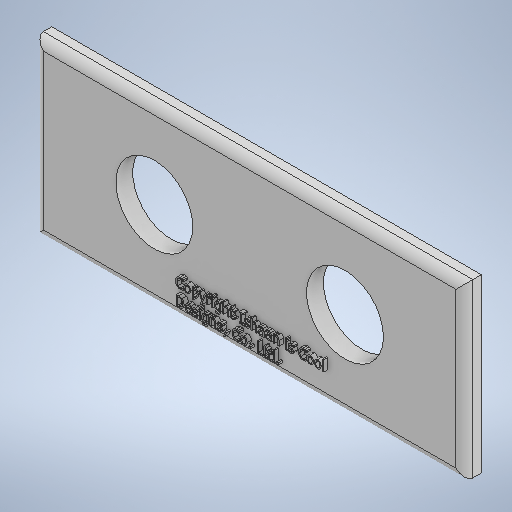
# Autodesk Inventor part: Hole Position Test Plate
Saved by Autodesk Inventor 2025.1 (Build 291241000, 241)
## iProperties
Created: 2024-12-13
Part Number: Hole Position Test Plate
Material: Generic
Document SubType Name: Modeling
Designer: ishaa
Density: 1 g/cm^3
Appearance: Default
Author: ishaa
Autodesk Inventor part; units mm, degrees
ref_plane "YZ Plane" through (0, 0, 0) normal (1, 0, 0) x (0, 1, 0)
ref_plane "XZ Plane" through (0, 0, 0) normal (0, 1, 0) x (-1, 0, 0)
ref_plane "XY Plane" through (0, 0, 0) normal (0, 0, 1) x (1, 0, 0)
sketch "Sketch1" plane through (0, 0, 0) normal (0, 0, 1) x (1, 0, 0)
  line L0 (-25.4, -10.16) -> (25.4, -10.16)
  line L1 (25.4, -10.16) -> (25.4, 10.16)
  line L2 (25.4, 10.16) -> (-25.4, 10.16)
  line L3 (-25.4, 10.16) -> (-25.4, -10.16)
  line L4 (-25.4, -10.16) -> (25.4, 10.16) construction
  line L5 (25.4, -10.16) -> (-25.4, 10.16) construction
  circle A0 centre (-11.276, 0) radius 4.55
  circle A1 centre (11.276, 0) radius 4.55
  line L6 (-11.276, 0) -> (11.276, 0) construction
  line L7 (0, 0) -> (0, 7.6048) construction
  line L8 (0, 15.995) -> (0, -21.9957) construction
  dimension "d0" = 50.8
  dimension "d1" = 20.32
  dimension "d2" = 9.1
  dimension "d3" = 9.1
  dimension "d4" = 22.552
  constraints: 18 end point, 3 midpoint, 3 vertical, 2 centre point, 2 horizontal, 2 parallel, 1 collinear, 1 perpendicular
  measures "d0" distance of L2.end L1.end
  measures "d1" distance of L1.end L0.end
  measures "d2" diameter of A0
  measures "d3" diameter of A1
  measures "d4" distance of L6.end L6.start
extrude "Extrusion1" add sketch "Sketch1" along normal blind 2
sketch "Sketch2" plane through (0, 0, 2) normal (0, 0, 1) x (1, 0, 0)
  line L0 (-8.3124, -5.381) -> (11.7699, -5.381) construction
  line L1 (11.7699, -5.381) -> (11.7699, -6.9151) construction
  line L2 (11.7699, -6.9151) -> (-8.3124, -6.9151) construction
  line L3 (-8.3124, -6.9151) -> (-8.3124, -5.381) construction
  spline S0 degree 2 poles (-7.7232, -6.6536) (-7.8397, -6.6536) (-8.0367, -6.575) (-8.1086, -6.4963) knots 0 0 0 1 2 2 2
  spline S1 degree 2 poles (-8.1086, -6.4963) (-8.1804, -6.4187) (-8.259, -6.1857) (-8.259, -6.0343) knots 0 0 0 1 2 2 2
  spline S2 degree 2 poles (-8.259, -6.0343) (-8.259, -5.8838) (-8.1823, -5.6606) (-8.1095, -5.578) knots 0 0 0 1 2 2 2
  spline S3 degree 2 poles (-8.1095, -5.578) (-8.0377, -5.4975) (-7.8416, -5.413) (-7.7203, -5.413) knots 0 0 0 1 2 2 2
  spline S4 degree 2 poles (-7.7203, -5.413) (-7.6601, -5.413) (-7.5543, -5.4305) (-7.5096, -5.4441) knots 0 0 0 1 2 2 2
  spline S5 degree 2 poles (-7.5096, -5.4441) (-7.4708, -5.4567) (-7.3902, -5.4926) (-7.3504, -5.514) knots 0 0 0 1 2 2 2
  line L4 (-7.3504, -5.514) -> (-7.3504, -5.7062)
  line L5 (-7.3504, -5.7062) -> (-7.3631, -5.7062)
  spline S6 degree 2 poles (-7.3631, -5.7062) (-7.3844, -5.6868) (-7.4504, -5.6324) (-7.498, -5.6062) knots 0 0 0 1 2 2 2
  spline S7 degree 2 poles (-7.498, -5.6062) (-7.5436, -5.581) (-7.6514, -5.5489) (-7.7213, -5.5489) knots 0 0 0 1 2 2 2
  spline S8 degree 2 poles (-7.7213, -5.5489) (-7.7979, -5.5489) (-7.9348, -5.612) (-7.9863, -5.6722) knots 0 0 0 1 2 2 2
  spline S9 degree 2 poles (-7.9863, -5.6722) (-8.0367, -5.7334) (-8.093, -5.9188) (-8.093, -6.0343) knots 0 0 0 1 2 2 2
  spline S10 degree 2 poles (-8.093, -6.0343) (-8.093, -6.1576) (-8.0338, -6.3352) (-7.9824, -6.3964) knots 0 0 0 1 2 2 2
  spline S11 degree 2 poles (-7.9824, -6.3964) (-7.9319, -6.4556) (-7.797, -6.5158) (-7.7213, -6.5158) knots 0 0 0 1 2 2 2
  spline S12 degree 2 poles (-7.7213, -6.5158) (-7.6523, -6.5158) (-7.5349, -6.4818) (-7.4893, -6.4565) knots 0 0 0 1 2 2 2
  spline S13 degree 2 poles (-7.4893, -6.4565) (-7.4456, -6.4313) (-7.3805, -6.3789) (-7.3621, -6.3604) knots 0 0 0 1 2 2 2
  line L6 (-7.3621, -6.3604) -> (-7.3504, -6.3604)
  line L7 (-7.3504, -6.3604) -> (-7.3504, -6.5507)
  spline S14 degree 2 poles (-7.3504, -6.5507) (-7.3902, -6.5692) (-7.4601, -6.6031) (-7.5096, -6.6187) knots 0 0 0 1 2 2 2
  spline S15 degree 2 poles (-7.5096, -6.6187) (-7.5621, -6.6361) (-7.6514, -6.6536) (-7.7232, -6.6536) knots 0 0 0 1 2 2 2
  spline S16 degree 2 poles (-6.4749, -6.1828) (-6.4749, -6.41) (-6.6933, -6.6575) (-6.8758, -6.6575) knots 0 0 0 1 2 2 2
  spline S17 degree 2 poles (-6.8758, -6.6575) (-7.0631, -6.6575) (-7.2776, -6.4022) (-7.2776, -6.1828) knots 0 0 0 1 2 2 2
  spline S18 degree 2 poles (-7.2776, -6.1828) (-7.2776, -5.9576) (-7.0563, -5.7081) (-6.8758, -5.7081) knots 0 0 0 1 2 2 2
  spline S19 degree 2 poles (-6.8758, -5.7081) (-6.6933, -5.7081) (-6.4749, -5.9566) (-6.4749, -6.1828) knots 0 0 0 1 2 2 2
  spline S20 degree 2 poles (-6.6311, -6.1828) (-6.6311, -6.0081) (-6.7583, -5.8382) (-6.8758, -5.8382) knots 0 0 0 1 2 2 2
  spline S21 degree 2 poles (-6.8758, -5.8382) (-6.9932, -5.8382) (-7.1214, -6.0081) (-7.1214, -6.1828) knots 0 0 0 1 2 2 2
  spline S22 degree 2 poles (-7.1214, -6.1828) (-7.1214, -6.3527) (-6.9932, -6.5274) (-6.8758, -6.5274) knots 0 0 0 1 2 2 2
  spline S23 degree 2 poles (-6.8758, -6.5274) (-6.7593, -6.5274) (-6.6311, -6.3556) (-6.6311, -6.1828) knots 0 0 0 1 2 2 2
  spline S24 degree 2 poles (-5.5663, -6.1585) (-5.5663, -6.3837) (-5.7808, -6.6497) (-5.9448, -6.6497) knots 0 0 0 1 2 2 2
  spline S25 degree 2 poles (-5.9448, -6.6497) (-6.0118, -6.6497) (-6.1147, -6.6187) (-6.1681, -6.5866) knots 0 0 0 1 2 2 2
  line L8 (-6.1681, -6.5866) -> (-6.1681, -6.9633)
  line L9 (-6.1681, -6.9633) -> (-6.3195, -6.9633)
  line L10 (-6.3195, -6.9633) -> (-6.3195, -5.7334)
  line L11 (-6.3195, -5.7334) -> (-6.1681, -5.7334)
  line L12 (-6.1681, -5.7334) -> (-6.1681, -5.8275)
  spline S26 degree 2 poles (-6.1681, -5.8275) (-6.1118, -5.7761) (-5.974, -5.7081) (-5.8934, -5.7081) knots 0 0 0 1 2 2 2
  spline S27 degree 2 poles (-5.8934, -5.7081) (-5.7391, -5.7081) (-5.5663, -5.9527) (-5.5663, -6.1585) knots 0 0 0 1 2 2 2
  spline S28 degree 2 poles (-5.7225, -6.176) (-5.7225, -6.0217) (-5.8206, -5.8518) (-5.9303, -5.8518) knots 0 0 0 1 2 2 2
  spline S29 degree 2 poles (-5.9303, -5.8518) (-5.9943, -5.8518) (-6.1147, -5.9091) (-6.1681, -5.9537) knots 0 0 0 1 2 2 2
  line L13 (-6.1681, -5.9537) -> (-6.1681, -6.4643)
  spline S30 degree 2 poles (-6.1681, -6.4643) (-6.1089, -6.4925) (-6.0244, -6.5138) (-5.9701, -6.5138) knots 0 0 0 1 2 2 2
  spline S31 degree 2 poles (-5.9701, -6.5138) (-5.8526, -6.5138) (-5.7225, -6.341) (-5.7225, -6.176) knots 0 0 0 1 2 2 2
  line L14 (-4.7033, -5.7334) -> (-5.1867, -6.9633)
  line L15 (-5.1867, -6.9633) -> (-5.3488, -6.9633)
  line L16 (-5.3488, -6.9633) -> (-5.1877, -6.5886)
  line L17 (-5.1877, -6.5886) -> (-5.5138, -5.7334)
  line L18 (-5.5138, -5.7334) -> (-5.3508, -5.7334)
  line L19 (-5.3508, -5.7334) -> (-5.1052, -6.3993)
  line L20 (-5.1052, -6.3993) -> (-4.8606, -5.7334)
  line L21 (-4.8606, -5.7334) -> (-4.7033, -5.7334)
  line L22 (-4.1121, -5.8955) -> (-4.1199, -5.8955)
  spline S32 degree 2 poles (-4.1199, -5.8955) (-4.1374, -5.8906) (-4.1752, -5.8887) (-4.2014, -5.8887) knots 0 0 0 1 2 2 2
  spline S33 degree 2 poles (-4.2014, -5.8887) (-4.2626, -5.8887) (-4.383, -5.9421) (-4.4373, -5.9945) knots 0 0 0 1 2 2 2
  line L23 (-4.4373, -5.9945) -> (-4.4373, -6.6322)
  line L24 (-4.4373, -6.6322) -> (-4.5888, -6.6322)
  line L25 (-4.5888, -6.6322) -> (-4.5888, -5.7334)
  line L26 (-4.5888, -5.7334) -> (-4.4373, -5.7334)
  line L27 (-4.4373, -5.7334) -> (-4.4373, -5.8673)
  spline S34 degree 2 poles (-4.4373, -5.8673) (-4.3548, -5.7935) (-4.2315, -5.7334) (-4.1733, -5.7334) knots 0 0 0 1 2 2 2
  spline S35 degree 2 poles (-4.1733, -5.7334) (-4.15, -5.7334) (-4.1267, -5.7353) (-4.1121, -5.7382) knots 0 0 0 1 2 2 2
  line L28 (-4.1121, -5.7382) -> (-4.1121, -5.8955)
  line L29 (-3.8403, -6.6322) -> (-3.9918, -6.6322)
  line L30 (-3.9918, -6.6322) -> (-3.9918, -5.7334)
  line L31 (-3.9918, -5.7334) -> (-3.8403, -5.7334)
  line L32 (-3.8403, -5.7334) -> (-3.8403, -6.6322)
  line L33 (-3.8297, -5.5839) -> (-4.0015, -5.5839)
  line L34 (-4.0015, -5.5839) -> (-4.0015, -5.4266)
  line L35 (-4.0015, -5.4266) -> (-3.8297, -5.4266)
  line L36 (-3.8297, -5.4266) -> (-3.8297, -5.5839)
  spline S36 degree 2 poles (-3.586, -6.7759) (-3.5705, -6.7827) (-3.5113, -6.8041) (-3.4734, -6.8128) knots 0 0 0 1 2 2 2
  spline S37 degree 2 poles (-3.4734, -6.8128) (-3.4317, -6.8235) (-3.3608, -6.8361) (-3.3191, -6.8361) knots 0 0 0 1 2 2 2
  spline S38 degree 2 poles (-3.3191, -6.8361) (-3.2492, -6.8361) (-3.1521, -6.7992) (-3.1249, -6.7662) knots 0 0 0 1 2 2 2
  spline S39 degree 2 poles (-3.1249, -6.7662) (-3.0987, -6.7332) (-3.0783, -6.6468) (-3.0783, -6.5915) knots 0 0 0 1 2 2 2
  line L37 (-3.0783, -6.5915) -> (-3.0783, -6.5128)
  spline S40 degree 2 poles (-3.0783, -6.5128) (-3.1395, -6.5662) (-3.2569, -6.6167) (-3.3453, -6.6167) knots 0 0 0 1 2 2 2
  spline S41 degree 2 poles (-3.3453, -6.6167) (-3.4986, -6.6167) (-3.6802, -6.3886) (-3.6802, -6.1741) knots 0 0 0 1 2 2 2
  spline S42 degree 2 poles (-3.6802, -6.1741) (-3.6802, -6.0624) (-3.6171, -5.8896) (-3.5646, -5.8285) knots 0 0 0 1 2 2 2
  spline S43 degree 2 poles (-3.5646, -5.8285) (-3.5142, -5.7712) (-3.3754, -5.7081) (-3.3016, -5.7081) knots 0 0 0 1 2 2 2
  spline S44 degree 2 poles (-3.3016, -5.7081) (-3.2317, -5.7081) (-3.1298, -5.7411) (-3.0783, -5.7712) knots 0 0 0 1 2 2 2
  line L38 (-3.0783, -5.7712) -> (-3.0696, -5.7334)
  line L39 (-3.0696, -5.7334) -> (-2.9269, -5.7334)
  line L40 (-2.9269, -5.7334) -> (-2.9269, -6.5294)
  spline S45 degree 2 poles (-2.9269, -6.5294) (-2.9269, -6.7584) (-3.1259, -6.972) (-3.3307, -6.972) knots 0 0 0 1 2 2 2
  spline S46 degree 2 poles (-3.3307, -6.972) (-3.3967, -6.972) (-3.5346, -6.9506) (-3.5938, -6.9332) knots 0 0 0 1 2 2 2
  line L41 (-3.5938, -6.9332) -> (-3.5938, -6.7759)
  line L42 (-3.5938, -6.7759) -> (-3.586, -6.7759)
  line L43 (-3.0783, -6.3886) -> (-3.0783, -5.8945)
  spline S47 degree 2 poles (-3.0783, -5.8945) (-3.1346, -5.8673) (-3.2297, -5.844) (-3.2773, -5.844) knots 0 0 0 1 2 2 2
  spline S48 degree 2 poles (-3.2773, -5.844) (-3.3919, -5.844) (-3.5239, -6.0129) (-3.5239, -6.1712) knots 0 0 0 1 2 2 2
  spline S49 degree 2 poles (-3.5239, -6.1712) (-3.5239, -6.3206) (-3.4239, -6.4769) (-3.3113, -6.4769) knots 0 0 0 1 2 2 2
  spline S50 degree 2 poles (-3.3113, -6.4769) (-3.2521, -6.4769) (-3.1278, -6.4303) (-3.0783, -6.3886) knots 0 0 0 1 2 2 2
  line L44 (-2.0018, -6.6322) -> (-2.1532, -6.6322)
  line L45 (-2.1532, -6.6322) -> (-2.1532, -6.1197)
  spline S51 degree 2 poles (-2.1532, -6.1197) (-2.1532, -6.0576) (-2.1649, -5.9508) (-2.1823, -5.9188) knots 0 0 0 1 2 2 2
  spline S52 degree 2 poles (-2.1823, -5.9188) (-2.2008, -5.8848) (-2.2668, -5.8518) (-2.3231, -5.8518) knots 0 0 0 1 2 2 2
  spline S53 degree 2 poles (-2.3231, -5.8518) (-2.3794, -5.8518) (-2.4988, -5.912) (-2.5561, -5.9605) knots 0 0 0 1 2 2 2
  line L46 (-2.5561, -5.9605) -> (-2.5561, -6.6322)
  line L47 (-2.5561, -6.6322) -> (-2.7075, -6.6322)
  line L48 (-2.7075, -6.6322) -> (-2.7075, -5.381)
  line L49 (-2.7075, -5.381) -> (-2.5561, -5.381)
  line L50 (-2.5561, -5.381) -> (-2.5561, -5.8333)
  spline S54 degree 2 poles (-2.5561, -5.8333) (-2.4881, -5.7722) (-2.3571, -5.7081) (-2.2833, -5.7081) knots 0 0 0 1 2 2 2
  spline S55 degree 2 poles (-2.2833, -5.7081) (-2.1513, -5.7081) (-2.0018, -5.8829) (-2.0018, -6.0488) knots 0 0 0 1 2 2 2
  line L51 (-2.0018, -6.0488) -> (-2.0018, -6.6322)
  spline S56 degree 2 poles (-1.5174, -6.6497) (-1.6407, -6.6497) (-1.7795, -6.509) (-1.7795, -6.3566) knots 0 0 0 1 2 2 2
  line L52 (-1.7795, -6.3566) -> (-1.7795, -5.8586)
  line L53 (-1.7795, -5.8586) -> (-1.8814, -5.8586)
  line L54 (-1.8814, -5.8586) -> (-1.8814, -5.7334)
  line L55 (-1.8814, -5.7334) -> (-1.7795, -5.7334)
  line L56 (-1.7795, -5.7334) -> (-1.7795, -5.4752)
  line L57 (-1.7795, -5.4752) -> (-1.6281, -5.4752)
  line L58 (-1.6281, -5.4752) -> (-1.6281, -5.7334)
  line L59 (-1.6281, -5.7334) -> (-1.3495, -5.7334)
  line L60 (-1.3495, -5.7334) -> (-1.3495, -5.8586)
  line L61 (-1.3495, -5.8586) -> (-1.6281, -5.8586)
  line L62 (-1.6281, -5.8586) -> (-1.6281, -6.2867)
  spline S57 degree 2 poles (-1.6281, -6.2867) (-1.6281, -6.3546) (-1.6232, -6.4294) (-1.6067, -6.4614) knots 0 0 0 1 2 2 2
  spline S58 degree 2 poles (-1.6067, -6.4614) (-1.5931, -6.4896) (-1.532, -6.5177) (-1.4795, -6.5177) knots 0 0 0 1 2 2 2
  spline S59 degree 2 poles (-1.4795, -6.5177) (-1.4427, -6.5177) (-1.3737, -6.4954) (-1.3582, -6.4886) knots 0 0 0 1 2 2 2
  line L63 (-1.3582, -6.4886) -> (-1.3495, -6.4886)
  line L64 (-1.3495, -6.4886) -> (-1.3495, -6.6245)
  spline S60 degree 2 poles (-1.3495, -6.6245) (-1.3922, -6.6361) (-1.4795, -6.6497) (-1.5174, -6.6497) knots 0 0 0 1 2 2 2
  line L65 (-0.2943, -6.6322) -> (-0.7583, -6.6322)
  line L66 (-0.7583, -6.6322) -> (-0.7583, -6.5099)
  line L67 (-0.7583, -6.5099) -> (-0.6059, -6.5099)
  line L68 (-0.6059, -6.5099) -> (-0.6059, -5.5567)
  line L69 (-0.6059, -5.5567) -> (-0.7583, -5.5567)
  line L70 (-0.7583, -5.5567) -> (-0.7583, -5.4344)
  line L71 (-0.7583, -5.4344) -> (-0.2943, -5.4344)
  line L72 (-0.2943, -5.4344) -> (-0.2943, -5.5567)
  line L73 (-0.2943, -5.5567) -> (-0.4467, -5.5567)
  line L74 (-0.4467, -5.5567) -> (-0.4467, -6.5099)
  line L75 (-0.4467, -6.5099) -> (-0.2943, -6.5099)
  line L76 (-0.2943, -6.5099) -> (-0.2943, -6.6322)
  spline S61 degree 2 poles (0.1338, -6.6536) (0.0435, -6.6536) (-0.1128, -6.6051) (-0.1642, -6.5779) knots 0 0 0 1 2 2 2
  line L77 (-0.1642, -6.5779) -> (-0.1642, -6.408)
  line L78 (-0.1642, -6.408) -> (-0.1565, -6.408)
  spline S62 degree 2 poles (-0.1565, -6.408) (-0.137, -6.4235) (-0.0846, -6.4604) (-0.0409, -6.4808) knots 0 0 0 1 2 2 2
  spline S63 degree 2 poles (-0.0409, -6.4808) (-0.0031, -6.4993) (0.0901, -6.5264) (0.1396, -6.5264) knots 0 0 0 1 2 2 2
  spline S64 degree 2 poles (0.1396, -6.5264) (0.1755, -6.5264) (0.258, -6.5099) (0.2774, -6.4963) knots 0 0 0 1 2 2 2
  spline S65 degree 2 poles (0.2774, -6.4963) (0.3056, -6.4779) (0.3308, -6.4362) (0.3308, -6.3935) knots 0 0 0 1 2 2 2
  spline S66 degree 2 poles (0.3308, -6.3935) (0.3308, -6.3401) (0.2726, -6.2847) (0.1979, -6.2663) knots 0 0 0 1 2 2 2
  spline S67 degree 2 poles (0.1979, -6.2663) (0.1687, -6.2595) (0.0755, -6.2401) (0.0357, -6.2294) knots 0 0 0 1 2 2 2
  spline S68 degree 2 poles (0.0357, -6.2294) (-0.0672, -6.1993) (-0.1603, -6.0751) (-0.1603, -5.9867) knots 0 0 0 1 2 2 2
  spline S69 degree 2 poles (-0.1603, -5.9867) (-0.1603, -5.8644) (0.0231, -5.712) (0.1746, -5.712) knots 0 0 0 1 2 2 2
  spline S70 degree 2 poles (0.1746, -5.712) (0.2493, -5.712) (0.4007, -5.7489) (0.4522, -5.777) knots 0 0 0 1 2 2 2
  line L79 (0.4522, -5.777) -> (0.4522, -5.9392)
  line L80 (0.4522, -5.9392) -> (0.4444, -5.9392)
  spline S71 degree 2 poles (0.4444, -5.9392) (0.3862, -5.8926) (0.2444, -5.8392) (0.1716, -5.8392) knots 0 0 0 1 2 2 2
  spline S72 degree 2 poles (0.1716, -5.8392) (0.0969, -5.8392) (-0.006, -5.9023) (-0.006, -5.9654) knots 0 0 0 1 2 2 2
  spline S73 degree 2 poles (-0.006, -5.9654) (-0.006, -6.0226) (0.0552, -6.078) (0.1231, -6.0954) knots 0 0 0 1 2 2 2
  spline S74 degree 2 poles (0.1231, -6.0954) (0.1561, -6.1042) (0.2396, -6.1217) (0.2852, -6.1323) knots 0 0 0 1 2 2 2
  spline S75 degree 2 poles (0.2852, -6.1323) (0.3842, -6.1576) (0.4852, -6.2731) (0.4852, -6.3731) knots 0 0 0 1 2 2 2
  spline S76 degree 2 poles (0.4852, -6.3731) (0.4852, -6.4313) (0.4396, -6.5342) (0.3949, -6.5721) knots 0 0 0 1 2 2 2
  spline S77 degree 2 poles (0.3949, -6.5721) (0.3473, -6.6119) (0.226, -6.6536) (0.1338, -6.6536) knots 0 0 0 1 2 2 2
  line L81 (1.3316, -6.6322) -> (1.1802, -6.6322)
  line L82 (1.1802, -6.6322) -> (1.1802, -6.1197)
  spline S78 degree 2 poles (1.1802, -6.1197) (1.1802, -6.0576) (1.1686, -5.9508) (1.1511, -5.9188) knots 0 0 0 1 2 2 2
  spline S79 degree 2 poles (1.1511, -5.9188) (1.1327, -5.8848) (1.0666, -5.8518) (1.0103, -5.8518) knots 0 0 0 1 2 2 2
  spline S80 degree 2 poles (1.0103, -5.8518) (0.954, -5.8518) (0.8346, -5.912) (0.7774, -5.9605) knots 0 0 0 1 2 2 2
  line L83 (0.7774, -5.9605) -> (0.7774, -6.6322)
  line L84 (0.7774, -6.6322) -> (0.6259, -6.6322)
  line L85 (0.6259, -6.6322) -> (0.6259, -5.381)
  line L86 (0.6259, -5.381) -> (0.7774, -5.381)
  line L87 (0.7774, -5.381) -> (0.7774, -5.8333)
  spline S81 degree 2 poles (0.7774, -5.8333) (0.8453, -5.7722) (0.9764, -5.7081) (1.0501, -5.7081) knots 0 0 0 1 2 2 2
  spline S82 degree 2 poles (1.0501, -5.7081) (1.1822, -5.7081) (1.3316, -5.8829) (1.3316, -6.0488) knots 0 0 0 1 2 2 2
  line L88 (1.3316, -6.0488) -> (1.3316, -6.6322)
  spline S83 degree 2 poles (2.0451, -6.5371) (2.0267, -6.5507) (1.9646, -6.5992) (1.9354, -6.6138) knots 0 0 0 1 2 2 2
  spline S84 degree 2 poles (1.9354, -6.6138) (1.8956, -6.6352) (1.8209, -6.6575) (1.7529, -6.6575) knots 0 0 0 1 2 2 2
  spline S85 degree 2 poles (1.7529, -6.6575) (1.6976, -6.6575) (1.5976, -6.6157) (1.5598, -6.5779) knots 0 0 0 1 2 2 2
  spline S86 degree 2 poles (1.5598, -6.5779) (1.5238, -6.541) (1.4802, -6.4323) (1.4802, -6.3721) knots 0 0 0 1 2 2 2
  spline S87 degree 2 poles (1.4802, -6.3721) (1.4802, -6.2789) (1.5588, -6.1469) (1.6442, -6.109) knots 0 0 0 1 2 2 2
  spline S88 degree 2 poles (1.6442, -6.109) (1.7199, -6.0741) (1.9257, -6.0479) (2.0451, -6.0411) knots 0 0 0 1 2 2 2
  line L89 (2.0451, -6.0411) -> (2.0451, -6.012)
  spline S89 degree 2 poles (2.0451, -6.012) (2.0451, -5.9595) (2.0131, -5.8945) (1.984, -5.8761) knots 0 0 0 1 2 2 2
  spline S90 degree 2 poles (1.984, -5.8761) (1.9548, -5.8576) (1.8714, -5.846) (1.8267, -5.846) knots 0 0 0 1 2 2 2
  spline S91 degree 2 poles (1.8267, -5.846) (1.7743, -5.846) (1.6326, -5.877) (1.5617, -5.9071) knots 0 0 0 1 2 2 2
  line L90 (1.5617, -5.9071) -> (1.553, -5.9071)
  line L91 (1.553, -5.9071) -> (1.553, -5.7528)
  spline S92 degree 2 poles (1.553, -5.7528) (1.5947, -5.7411) (1.751, -5.712) (1.8277, -5.712) knots 0 0 0 1 2 2 2
  spline S93 degree 2 poles (1.8277, -5.712) (1.9209, -5.712) (2.048, -5.7411) (2.0985, -5.779) knots 0 0 0 1 2 2 2
  spline S94 degree 2 poles (2.0985, -5.779) (2.148, -5.8159) (2.1966, -5.9333) (2.1966, -6.0178) knots 0 0 0 1 2 2 2
  line L92 (2.1966, -6.0178) -> (2.1966, -6.6322)
  line L93 (2.1966, -6.6322) -> (2.0451, -6.6322)
  line L94 (2.0451, -6.6322) -> (2.0451, -6.5371)
  line L95 (2.0451, -6.4109) -> (2.0451, -6.1615)
  spline S95 degree 2 poles (2.0451, -6.1615) (1.9908, -6.1663) (1.8267, -6.1828) (1.7753, -6.1983) knots 0 0 0 1 2 2 2
  spline S96 degree 2 poles (1.7753, -6.1983) (1.7151, -6.2168) (1.6365, -6.2935) (1.6365, -6.3614) knots 0 0 0 1 2 2 2
  spline S97 degree 2 poles (1.6365, -6.3614) (1.6365, -6.4391) (1.7238, -6.5177) (1.8073, -6.5177) knots 0 0 0 1 2 2 2
  spline S98 degree 2 poles (1.8073, -6.5177) (1.8782, -6.5177) (1.9946, -6.4565) (2.0451, -6.4109) knots 0 0 0 1 2 2 2
  spline S99 degree 2 poles (2.91, -6.5371) (2.8916, -6.5507) (2.8295, -6.5992) (2.8003, -6.6138) knots 0 0 0 1 2 2 2
  spline S100 degree 2 poles (2.8003, -6.6138) (2.7605, -6.6352) (2.6858, -6.6575) (2.6178, -6.6575) knots 0 0 0 1 2 2 2
  spline S101 degree 2 poles (2.6178, -6.6575) (2.5625, -6.6575) (2.4625, -6.6157) (2.4247, -6.5779) knots 0 0 0 1 2 2 2
  spline S102 degree 2 poles (2.4247, -6.5779) (2.3888, -6.541) (2.3451, -6.4323) (2.3451, -6.3721) knots 0 0 0 1 2 2 2
  spline S103 degree 2 poles (2.3451, -6.3721) (2.3451, -6.2789) (2.4237, -6.1469) (2.5091, -6.109) knots 0 0 0 1 2 2 2
  spline S104 degree 2 poles (2.5091, -6.109) (2.5848, -6.0741) (2.7906, -6.0479) (2.91, -6.0411) knots 0 0 0 1 2 2 2
  line L96 (2.91, -6.0411) -> (2.91, -6.012)
  spline S105 degree 2 poles (2.91, -6.012) (2.91, -5.9595) (2.878, -5.8945) (2.8489, -5.8761) knots 0 0 0 1 2 2 2
  spline S106 degree 2 poles (2.8489, -5.8761) (2.8198, -5.8576) (2.7363, -5.846) (2.6916, -5.846) knots 0 0 0 1 2 2 2
  spline S107 degree 2 poles (2.6916, -5.846) (2.6392, -5.846) (2.4975, -5.877) (2.4266, -5.9071) knots 0 0 0 1 2 2 2
  line L97 (2.4266, -5.9071) -> (2.4179, -5.9071)
  line L98 (2.4179, -5.9071) -> (2.4179, -5.7528)
  spline S108 degree 2 poles (2.4179, -5.7528) (2.4596, -5.7411) (2.6159, -5.712) (2.6926, -5.712) knots 0 0 0 1 2 2 2
  spline S109 degree 2 poles (2.6926, -5.712) (2.7858, -5.712) (2.9129, -5.7411) (2.9634, -5.779) knots 0 0 0 1 2 2 2
  spline S110 degree 2 poles (2.9634, -5.779) (3.0129, -5.8159) (3.0615, -5.9333) (3.0615, -6.0178) knots 0 0 0 1 2 2 2
  line L99 (3.0615, -6.0178) -> (3.0615, -6.6322)
  line L100 (3.0615, -6.6322) -> (2.91, -6.6322)
  line L101 (2.91, -6.6322) -> (2.91, -6.5371)
  line L102 (2.91, -6.4109) -> (2.91, -6.1615)
  spline S111 degree 2 poles (2.91, -6.1615) (2.8557, -6.1663) (2.6916, -6.1828) (2.6402, -6.1983) knots 0 0 0 1 2 2 2
  spline S112 degree 2 poles (2.6402, -6.1983) (2.58, -6.2168) (2.5014, -6.2935) (2.5014, -6.3614) knots 0 0 0 1 2 2 2
  spline S113 degree 2 poles (2.5014, -6.3614) (2.5014, -6.4391) (2.5887, -6.5177) (2.6722, -6.5177) knots 0 0 0 1 2 2 2
  spline S114 degree 2 poles (2.6722, -6.5177) (2.7431, -6.5177) (2.8596, -6.4565) (2.91, -6.4109) knots 0 0 0 1 2 2 2
  line L103 (3.9798, -6.6322) -> (3.8283, -6.6322)
  line L104 (3.8283, -6.6322) -> (3.8283, -6.1197)
  spline S115 degree 2 poles (3.8283, -6.1197) (3.8283, -6.0576) (3.8167, -5.9508) (3.7992, -5.9188) knots 0 0 0 1 2 2 2
  spline S116 degree 2 poles (3.7992, -5.9188) (3.7808, -5.8848) (3.7148, -5.8518) (3.6585, -5.8518) knots 0 0 0 1 2 2 2
  spline S117 degree 2 poles (3.6585, -5.8518) (3.6022, -5.8518) (3.4828, -5.912) (3.4255, -5.9605) knots 0 0 0 1 2 2 2
  line L105 (3.4255, -5.9605) -> (3.4255, -6.6322)
  line L106 (3.4255, -6.6322) -> (3.2741, -6.6322)
  line L107 (3.2741, -6.6322) -> (3.2741, -5.7334)
  line L108 (3.2741, -5.7334) -> (3.4255, -5.7334)
  line L109 (3.4255, -5.7334) -> (3.4255, -5.8333)
  spline S118 degree 2 poles (3.4255, -5.8333) (3.4934, -5.7722) (3.6245, -5.7081) (3.6983, -5.7081) knots 0 0 0 1 2 2 2
  spline S119 degree 2 poles (3.6983, -5.7081) (3.8303, -5.7081) (3.9798, -5.8829) (3.9798, -6.0488) knots 0 0 0 1 2 2 2
  line L110 (3.9798, -6.0488) -> (3.9798, -6.6322)
  line L111 (4.8612, -6.6322) -> (4.7097, -6.6322)
  line L112 (4.7097, -6.6322) -> (4.7097, -5.7334)
  line L113 (4.7097, -5.7334) -> (4.8612, -5.7334)
  line L114 (4.8612, -5.7334) -> (4.8612, -6.6322)
  line L115 (4.8718, -5.5839) -> (4.7, -5.5839)
  line L116 (4.7, -5.5839) -> (4.7, -5.4266)
  line L117 (4.7, -5.4266) -> (4.8718, -5.4266)
  line L118 (4.8718, -5.4266) -> (4.8718, -5.5839)
  spline S120 degree 2 poles (5.3261, -6.6536) (5.2359, -6.6536) (5.0796, -6.6051) (5.0281, -6.5779) knots 0 0 0 1 2 2 2
  line L119 (5.0281, -6.5779) -> (5.0281, -6.408)
  line L120 (5.0281, -6.408) -> (5.0359, -6.408)
  spline S121 degree 2 poles (5.0359, -6.408) (5.0553, -6.4235) (5.1077, -6.4604) (5.1514, -6.4808) knots 0 0 0 1 2 2 2
  spline S122 degree 2 poles (5.1514, -6.4808) (5.1893, -6.4993) (5.2825, -6.5264) (5.332, -6.5264) knots 0 0 0 1 2 2 2
  spline S123 degree 2 poles (5.332, -6.5264) (5.3679, -6.5264) (5.4504, -6.5099) (5.4698, -6.4963) knots 0 0 0 1 2 2 2
  spline S124 degree 2 poles (5.4698, -6.4963) (5.498, -6.4779) (5.5232, -6.4362) (5.5232, -6.3935) knots 0 0 0 1 2 2 2
  spline S125 degree 2 poles (5.5232, -6.3935) (5.5232, -6.3401) (5.465, -6.2847) (5.3902, -6.2663) knots 0 0 0 1 2 2 2
  spline S126 degree 2 poles (5.3902, -6.2663) (5.3611, -6.2595) (5.2679, -6.2401) (5.2281, -6.2294) knots 0 0 0 1 2 2 2
  spline S127 degree 2 poles (5.2281, -6.2294) (5.1252, -6.1993) (5.032, -6.0751) (5.032, -5.9867) knots 0 0 0 1 2 2 2
  spline S128 degree 2 poles (5.032, -5.9867) (5.032, -5.8644) (5.2155, -5.712) (5.3669, -5.712) knots 0 0 0 1 2 2 2
  spline S129 degree 2 poles (5.3669, -5.712) (5.4417, -5.712) (5.5931, -5.7489) (5.6445, -5.777) knots 0 0 0 1 2 2 2
  line L121 (5.6445, -5.777) -> (5.6445, -5.9392)
  line L122 (5.6445, -5.9392) -> (5.6368, -5.9392)
  spline S130 degree 2 poles (5.6368, -5.9392) (5.5785, -5.8926) (5.4368, -5.8392) (5.364, -5.8392) knots 0 0 0 1 2 2 2
  spline S131 degree 2 poles (5.364, -5.8392) (5.2893, -5.8392) (5.1864, -5.9023) (5.1864, -5.9654) knots 0 0 0 1 2 2 2
  spline S132 degree 2 poles (5.1864, -5.9654) (5.1864, -6.0226) (5.2475, -6.078) (5.3155, -6.0954) knots 0 0 0 1 2 2 2
  spline S133 degree 2 poles (5.3155, -6.0954) (5.3485, -6.1042) (5.432, -6.1217) (5.4776, -6.1323) knots 0 0 0 1 2 2 2
  spline S134 degree 2 poles (5.4776, -6.1323) (5.5766, -6.1576) (5.6775, -6.2731) (5.6775, -6.3731) knots 0 0 0 1 2 2 2
  spline S135 degree 2 poles (5.6775, -6.3731) (5.6775, -6.4313) (5.6319, -6.5342) (5.5873, -6.5721) knots 0 0 0 1 2 2 2
  spline S136 degree 2 poles (5.5873, -6.5721) (5.5397, -6.6119) (5.4184, -6.6536) (5.3261, -6.6536) knots 0 0 0 1 2 2 2
  spline S137 degree 2 poles (6.8123, -6.6536) (6.6958, -6.6536) (6.4988, -6.575) (6.4269, -6.4963) knots 0 0 0 1 2 2 2
  spline S138 degree 2 poles (6.4269, -6.4963) (6.3551, -6.4187) (6.2765, -6.1857) (6.2765, -6.0343) knots 0 0 0 1 2 2 2
  spline S139 degree 2 poles (6.2765, -6.0343) (6.2765, -5.8838) (6.3532, -5.6606) (6.426, -5.578) knots 0 0 0 1 2 2 2
  spline S140 degree 2 poles (6.426, -5.578) (6.4978, -5.4975) (6.6939, -5.413) (6.8152, -5.413) knots 0 0 0 1 2 2 2
  spline S141 degree 2 poles (6.8152, -5.413) (6.8754, -5.413) (6.9812, -5.4305) (7.0259, -5.4441) knots 0 0 0 1 2 2 2
  spline S142 degree 2 poles (7.0259, -5.4441) (7.0647, -5.4567) (7.1453, -5.4926) (7.1851, -5.514) knots 0 0 0 1 2 2 2
  line L123 (7.1851, -5.514) -> (7.1851, -5.7062)
  line L124 (7.1851, -5.7062) -> (7.1724, -5.7062)
  spline S143 degree 2 poles (7.1724, -5.7062) (7.1511, -5.6868) (7.0851, -5.6324) (7.0375, -5.6062) knots 0 0 0 1 2 2 2
  spline S144 degree 2 poles (7.0375, -5.6062) (6.9919, -5.581) (6.8841, -5.5489) (6.8143, -5.5489) knots 0 0 0 1 2 2 2
  spline S145 degree 2 poles (6.8143, -5.5489) (6.7376, -5.5489) (6.6007, -5.612) (6.5492, -5.6722) knots 0 0 0 1 2 2 2
  spline S146 degree 2 poles (6.5492, -5.6722) (6.4988, -5.7334) (6.4425, -5.9188) (6.4425, -6.0343) knots 0 0 0 1 2 2 2
  spline S147 degree 2 poles (6.4425, -6.0343) (6.4425, -6.1576) (6.5017, -6.3352) (6.5531, -6.3964) knots 0 0 0 1 2 2 2
  spline S148 degree 2 poles (6.5531, -6.3964) (6.6036, -6.4556) (6.7385, -6.5158) (6.8143, -6.5158) knots 0 0 0 1 2 2 2
  spline S149 degree 2 poles (6.8143, -6.5158) (6.8832, -6.5158) (7.0006, -6.4818) (7.0463, -6.4565) knots 0 0 0 1 2 2 2
  spline S150 degree 2 poles (7.0463, -6.4565) (7.0899, -6.4313) (7.155, -6.3789) (7.1734, -6.3604) knots 0 0 0 1 2 2 2
  line L125 (7.1734, -6.3604) -> (7.1851, -6.3604)
  line L126 (7.1851, -6.3604) -> (7.1851, -6.5507)
  spline S151 degree 2 poles (7.1851, -6.5507) (7.1453, -6.5692) (7.0754, -6.6031) (7.0259, -6.6187) knots 0 0 0 1 2 2 2
  spline S152 degree 2 poles (7.0259, -6.6187) (6.9735, -6.6361) (6.8841, -6.6536) (6.8123, -6.6536) knots 0 0 0 1 2 2 2
  spline S153 degree 2 poles (8.0607, -6.1828) (8.0607, -6.41) (7.8422, -6.6575) (7.6597, -6.6575) knots 0 0 0 1 2 2 2
  spline S154 degree 2 poles (7.6597, -6.6575) (7.4724, -6.6575) (7.2579, -6.4022) (7.2579, -6.1828) knots 0 0 0 1 2 2 2
  spline S155 degree 2 poles (7.2579, -6.1828) (7.2579, -5.9576) (7.4792, -5.7081) (7.6597, -5.7081) knots 0 0 0 1 2 2 2
  spline S156 degree 2 poles (7.6597, -5.7081) (7.8422, -5.7081) (8.0607, -5.9566) (8.0607, -6.1828) knots 0 0 0 1 2 2 2
  spline S157 degree 2 poles (7.9044, -6.1828) (7.9044, -6.0081) (7.7772, -5.8382) (7.6597, -5.8382) knots 0 0 0 1 2 2 2
  spline S158 degree 2 poles (7.6597, -5.8382) (7.5423, -5.8382) (7.4142, -6.0081) (7.4142, -6.1828) knots 0 0 0 1 2 2 2
  spline S159 degree 2 poles (7.4142, -6.1828) (7.4142, -6.3527) (7.5423, -6.5274) (7.6597, -6.5274) knots 0 0 0 1 2 2 2
  spline S160 degree 2 poles (7.6597, -6.5274) (7.7762, -6.5274) (7.9044, -6.3556) (7.9044, -6.1828) knots 0 0 0 1 2 2 2
  spline S161 degree 2 poles (8.9547, -6.1828) (8.9547, -6.41) (8.7363, -6.6575) (8.5538, -6.6575) knots 0 0 0 1 2 2 2
  spline S162 degree 2 poles (8.5538, -6.6575) (8.3664, -6.6575) (8.1519, -6.4022) (8.1519, -6.1828) knots 0 0 0 1 2 2 2
  spline S163 degree 2 poles (8.1519, -6.1828) (8.1519, -5.9576) (8.3732, -5.7081) (8.5538, -5.7081) knots 0 0 0 1 2 2 2
  spline S164 degree 2 poles (8.5538, -5.7081) (8.7363, -5.7081) (8.9547, -5.9566) (8.9547, -6.1828) knots 0 0 0 1 2 2 2
  spline S165 degree 2 poles (8.7984, -6.1828) (8.7984, -6.0081) (8.6712, -5.8382) (8.5538, -5.8382) knots 0 0 0 1 2 2 2
  spline S166 degree 2 poles (8.5538, -5.8382) (8.4363, -5.8382) (8.3082, -6.0081) (8.3082, -6.1828) knots 0 0 0 1 2 2 2
  spline S167 degree 2 poles (8.3082, -6.1828) (8.3082, -6.3527) (8.4363, -6.5274) (8.5538, -6.5274) knots 0 0 0 1 2 2 2
  spline S168 degree 2 poles (8.5538, -6.5274) (8.6703, -6.5274) (8.7984, -6.3556) (8.7984, -6.1828) knots 0 0 0 1 2 2 2
  line L127 (9.2643, -6.6322) -> (9.1129, -6.6322)
  line L128 (9.1129, -6.6322) -> (9.1129, -5.381)
  line L129 (9.1129, -5.381) -> (9.2643, -5.381)
  line L130 (9.2643, -5.381) -> (9.2643, -6.6322)
  spline S169 degree 2 poles (-7.2466, -8.0065) (-7.2466, -8.1706) (-7.3796, -8.4346) (-7.4912, -8.5084) knots 0 0 0 1 2 2 2
  spline S170 degree 2 poles (-7.4912, -8.5084) (-7.5824, -8.5657) (-7.7698, -8.6045) (-7.9154, -8.6045) knots 0 0 0 1 2 2 2
  line L131 (-7.9154, -8.6045) -> (-8.1911, -8.6045)
  line L132 (-8.1911, -8.6045) -> (-8.1911, -7.4066)
  line L133 (-8.1911, -7.4066) -> (-7.9183, -7.4066)
  spline S171 degree 2 poles (-7.9183, -7.4066) (-7.7494, -7.4066) (-7.5572, -7.4571) (-7.4893, -7.5018) knots 0 0 0 1 2 2 2
  spline S172 degree 2 poles (-7.4893, -7.5018) (-7.3737, -7.5785) (-7.2466, -7.8318) (-7.2466, -8.0065) knots 0 0 0 1 2 2 2
  spline S173 degree 2 poles (-7.4126, -8.0046) (-7.4126, -7.8668) (-7.5038, -7.6716) (-7.5941, -7.6163) knots 0 0 0 1 2 2 2
  spline S174 degree 2 poles (-7.5941, -7.6163) (-7.6582, -7.5785) (-7.8028, -7.5445) (-7.9105, -7.5445) knots 0 0 0 1 2 2 2
  line L134 (-7.9105, -7.5445) -> (-8.0319, -7.5445)
  line L135 (-8.0319, -7.5445) -> (-8.0319, -8.4667)
  line L136 (-8.0319, -8.4667) -> (-7.9105, -8.4667)
  spline S175 degree 2 poles (-7.9105, -8.4667) (-7.8047, -8.4667) (-7.6446, -8.4327) (-7.5795, -8.3871) knots 0 0 0 1 2 2 2
  spline S176 degree 2 poles (-7.5795, -8.3871) (-7.496, -8.3308) (-7.4126, -8.1444) (-7.4126, -8.0046) knots 0 0 0 1 2 2 2
  spline S177 degree 2 poles (-6.6952, -8.6249) (-6.9107, -8.6249) (-7.1476, -8.3832) (-7.1476, -8.1599) knots 0 0 0 1 2 2 2
  spline S178 degree 2 poles (-7.1476, -8.1599) (-7.1476, -7.9405) (-6.9175, -7.6804) (-6.7321, -7.6804) knots 0 0 0 1 2 2 2
  spline S179 degree 2 poles (-6.7321, -7.6804) (-6.6486, -7.6804) (-6.5195, -7.7289) (-6.4719, -7.7804) knots 0 0 0 1 2 2 2
  spline S180 degree 2 poles (-6.4719, -7.7804) (-6.4234, -7.8318) (-6.372, -7.9803) (-6.372, -8.0881) knots 0 0 0 1 2 2 2
  line L137 (-6.372, -8.0881) -> (-6.372, -8.1706)
  line L138 (-6.372, -8.1706) -> (-6.9942, -8.1706)
  spline S181 degree 2 poles (-6.9942, -8.1706) (-6.9942, -8.3269) (-6.8369, -8.4929) (-6.6971, -8.4929) knots 0 0 0 1 2 2 2
  spline S182 degree 2 poles (-6.6971, -8.4929) (-6.6476, -8.4929) (-6.5515, -8.4705) (-6.5127, -8.4531) knots 0 0 0 1 2 2 2
  spline S183 degree 2 poles (-6.5127, -8.4531) (-6.4719, -8.4337) (-6.4156, -8.3997) (-6.3972, -8.3841) knots 0 0 0 1 2 2 2
  line L139 (-6.3972, -8.3841) -> (-6.3885, -8.3841)
  line L140 (-6.3885, -8.3841) -> (-6.3885, -8.5492)
  spline S184 degree 2 poles (-6.3885, -8.5492) (-6.4147, -8.5598) (-6.4943, -8.5909) (-6.5253, -8.5996) knots 0 0 0 1 2 2 2
  spline S185 degree 2 poles (-6.5253, -8.5996) (-6.569, -8.6123) (-6.6408, -8.6249) (-6.6952, -8.6249) knots 0 0 0 1 2 2 2
  spline S186 degree 2 poles (-6.5195, -8.0551) (-6.5214, -7.9939) (-6.5467, -7.9046) (-6.571, -7.8745) knots 0 0 0 1 2 2 2
  spline S187 degree 2 poles (-6.571, -7.8745) (-6.5972, -7.8405) (-6.6797, -7.8046) (-6.7408, -7.8046) knots 0 0 0 1 2 2 2
  spline S188 degree 2 poles (-6.7408, -7.8046) (-6.801, -7.8046) (-6.8855, -7.8405) (-6.9204, -7.8755) knots 0 0 0 1 2 2 2
  spline S189 degree 2 poles (-6.9204, -7.8755) (-6.9544, -7.9114) (-6.9893, -7.9978) (-6.9942, -8.0551) knots 0 0 0 1 2 2 2
  line L141 (-6.9942, -8.0551) -> (-6.5195, -8.0551)
  spline S190 degree 2 poles (-5.9759, -8.6259) (-6.0662, -8.6259) (-6.2225, -8.5773) (-6.2739, -8.5501) knots 0 0 0 1 2 2 2
  line L142 (-6.2739, -8.5501) -> (-6.2739, -8.3803)
  line L143 (-6.2739, -8.3803) -> (-6.2662, -8.3803)
  spline S191 degree 2 poles (-6.2662, -8.3803) (-6.2467, -8.3958) (-6.1943, -8.4327) (-6.1506, -8.4531) knots 0 0 0 1 2 2 2
  spline S192 degree 2 poles (-6.1506, -8.4531) (-6.1128, -8.4715) (-6.0196, -8.4987) (-5.9701, -8.4987) knots 0 0 0 1 2 2 2
  spline S193 degree 2 poles (-5.9701, -8.4987) (-5.9342, -8.4987) (-5.8517, -8.4822) (-5.8322, -8.4686) knots 0 0 0 1 2 2 2
  spline S194 degree 2 poles (-5.8322, -8.4686) (-5.8041, -8.4502) (-5.7789, -8.4084) (-5.7789, -8.3657) knots 0 0 0 1 2 2 2
  spline S195 degree 2 poles (-5.7789, -8.3657) (-5.7789, -8.3123) (-5.8371, -8.257) (-5.9118, -8.2385) knots 0 0 0 1 2 2 2
  spline S196 degree 2 poles (-5.9118, -8.2385) (-5.941, -8.2317) (-6.0341, -8.2123) (-6.0739, -8.2017) knots 0 0 0 1 2 2 2
  spline S197 degree 2 poles (-6.0739, -8.2017) (-6.1768, -8.1716) (-6.27, -8.0473) (-6.27, -7.959) knots 0 0 0 1 2 2 2
  spline S198 degree 2 poles (-6.27, -7.959) (-6.27, -7.8367) (-6.0866, -7.6843) (-5.9351, -7.6843) knots 0 0 0 1 2 2 2
  spline S199 degree 2 poles (-5.9351, -7.6843) (-5.8604, -7.6843) (-5.709, -7.7211) (-5.6575, -7.7493) knots 0 0 0 1 2 2 2
  line L144 (-5.6575, -7.7493) -> (-5.6575, -7.9114)
  line L145 (-5.6575, -7.9114) -> (-5.6653, -7.9114)
  spline S200 degree 2 poles (-5.6653, -7.9114) (-5.7235, -7.8648) (-5.8652, -7.8114) (-5.938, -7.8114) knots 0 0 0 1 2 2 2
  spline S201 degree 2 poles (-5.938, -7.8114) (-6.0128, -7.8114) (-6.1157, -7.8745) (-6.1157, -7.9376) knots 0 0 0 1 2 2 2
  spline S202 degree 2 poles (-6.1157, -7.9376) (-6.1157, -7.9949) (-6.0545, -8.0502) (-5.9866, -8.0677) knots 0 0 0 1 2 2 2
  spline S203 degree 2 poles (-5.9866, -8.0677) (-5.9536, -8.0764) (-5.8701, -8.0939) (-5.8245, -8.1046) knots 0 0 0 1 2 2 2
  spline S204 degree 2 poles (-5.8245, -8.1046) (-5.7255, -8.1298) (-5.6245, -8.2453) (-5.6245, -8.3453) knots 0 0 0 1 2 2 2
  spline S205 degree 2 poles (-5.6245, -8.3453) (-5.6245, -8.4036) (-5.6701, -8.5065) (-5.7148, -8.5443) knots 0 0 0 1 2 2 2
  spline S206 degree 2 poles (-5.7148, -8.5443) (-5.7623, -8.5841) (-5.8837, -8.6259) (-5.9759, -8.6259) knots 0 0 0 1 2 2 2
  line L146 (-5.3294, -8.6045) -> (-5.4808, -8.6045)
  line L147 (-5.4808, -8.6045) -> (-5.4808, -7.7056)
  line L148 (-5.4808, -7.7056) -> (-5.3294, -7.7056)
  line L149 (-5.3294, -7.7056) -> (-5.3294, -8.6045)
  line L150 (-5.3187, -7.5561) -> (-5.4905, -7.5561)
  line L151 (-5.4905, -7.5561) -> (-5.4905, -7.3989)
  line L152 (-5.4905, -7.3989) -> (-5.3187, -7.3989)
  line L153 (-5.3187, -7.3989) -> (-5.3187, -7.5561)
  spline S207 degree 2 poles (-5.0751, -8.7482) (-5.0595, -8.755) (-5.0003, -8.7763) (-4.9625, -8.7851) knots 0 0 0 1 2 2 2
  spline S208 degree 2 poles (-4.9625, -8.7851) (-4.9207, -8.7957) (-4.8499, -8.8083) (-4.8081, -8.8083) knots 0 0 0 1 2 2 2
  spline S209 degree 2 poles (-4.8081, -8.8083) (-4.7382, -8.8083) (-4.6412, -8.7715) (-4.614, -8.7385) knots 0 0 0 1 2 2 2
  spline S210 degree 2 poles (-4.614, -8.7385) (-4.5878, -8.7055) (-4.5674, -8.6191) (-4.5674, -8.5637) knots 0 0 0 1 2 2 2
  line L154 (-4.5674, -8.5637) -> (-4.5674, -8.4851)
  spline S211 degree 2 poles (-4.5674, -8.4851) (-4.6286, -8.5385) (-4.746, -8.589) (-4.8343, -8.589) knots 0 0 0 1 2 2 2
  spline S212 degree 2 poles (-4.8343, -8.589) (-4.9877, -8.589) (-5.1692, -8.3608) (-5.1692, -8.1463) knots 0 0 0 1 2 2 2
  spline S213 degree 2 poles (-5.1692, -8.1463) (-5.1692, -8.0347) (-5.1061, -7.8619) (-5.0537, -7.8007) knots 0 0 0 1 2 2 2
  spline S214 degree 2 poles (-5.0537, -7.8007) (-5.0032, -7.7435) (-4.8644, -7.6804) (-4.7907, -7.6804) knots 0 0 0 1 2 2 2
  spline S215 degree 2 poles (-4.7907, -7.6804) (-4.7208, -7.6804) (-4.6188, -7.7134) (-4.5674, -7.7435) knots 0 0 0 1 2 2 2
  line L155 (-4.5674, -7.7435) -> (-4.5587, -7.7056)
  line L156 (-4.5587, -7.7056) -> (-4.416, -7.7056)
  line L157 (-4.416, -7.7056) -> (-4.416, -8.5016)
  spline S216 degree 2 poles (-4.416, -8.5016) (-4.416, -8.7307) (-4.615, -8.9442) (-4.8198, -8.9442) knots 0 0 0 1 2 2 2
  spline S217 degree 2 poles (-4.8198, -8.9442) (-4.8858, -8.9442) (-5.0236, -8.9229) (-5.0828, -8.9054) knots 0 0 0 1 2 2 2
  line L158 (-5.0828, -8.9054) -> (-5.0828, -8.7482)
  line L159 (-5.0828, -8.7482) -> (-5.0751, -8.7482)
  line L160 (-4.5674, -8.3608) -> (-4.5674, -7.8668)
  spline S218 degree 2 poles (-4.5674, -7.8668) (-4.6237, -7.8396) (-4.7188, -7.8163) (-4.7664, -7.8163) knots 0 0 0 1 2 2 2
  spline S219 degree 2 poles (-4.7664, -7.8163) (-4.8809, -7.8163) (-5.013, -7.9852) (-5.013, -8.1434) knots 0 0 0 1 2 2 2
  spline S220 degree 2 poles (-5.013, -8.1434) (-5.013, -8.2929) (-4.913, -8.4492) (-4.8004, -8.4492) knots 0 0 0 1 2 2 2
  spline S221 degree 2 poles (-4.8004, -8.4492) (-4.7412, -8.4492) (-4.6169, -8.4026) (-4.5674, -8.3608) knots 0 0 0 1 2 2 2
  line L161 (-3.4909, -8.6045) -> (-3.6423, -8.6045)
  line L162 (-3.6423, -8.6045) -> (-3.6423, -8.092)
  spline S222 degree 2 poles (-3.6423, -8.092) (-3.6423, -8.0298) (-3.654, -7.9231) (-3.6714, -7.891) knots 0 0 0 1 2 2 2
  spline S223 degree 2 poles (-3.6714, -7.891) (-3.6899, -7.857) (-3.7559, -7.824) (-3.8122, -7.824) knots 0 0 0 1 2 2 2
  spline S224 degree 2 poles (-3.8122, -7.824) (-3.8685, -7.824) (-3.9879, -7.8842) (-4.0452, -7.9328) knots 0 0 0 1 2 2 2
  line L163 (-4.0452, -7.9328) -> (-4.0452, -8.6045)
  line L164 (-4.0452, -8.6045) -> (-4.1966, -8.6045)
  line L165 (-4.1966, -8.6045) -> (-4.1966, -7.7056)
  line L166 (-4.1966, -7.7056) -> (-4.0452, -7.7056)
  line L167 (-4.0452, -7.7056) -> (-4.0452, -7.8056)
  spline S225 degree 2 poles (-4.0452, -7.8056) (-3.9772, -7.7444) (-3.8462, -7.6804) (-3.7724, -7.6804) knots 0 0 0 1 2 2 2
  spline S226 degree 2 poles (-3.7724, -7.6804) (-3.6404, -7.6804) (-3.4909, -7.8551) (-3.4909, -8.0211) knots 0 0 0 1 2 2 2
  line L168 (-3.4909, -8.0211) -> (-3.4909, -8.6045)
  spline S227 degree 2 poles (-3.0356, -8.6259) (-3.1259, -8.6259) (-3.2822, -8.5773) (-3.3336, -8.5501) knots 0 0 0 1 2 2 2
  line L169 (-3.3336, -8.5501) -> (-3.3336, -8.3803)
  line L170 (-3.3336, -8.3803) -> (-3.3259, -8.3803)
  spline S228 degree 2 poles (-3.3259, -8.3803) (-3.3064, -8.3958) (-3.254, -8.4327) (-3.2103, -8.4531) knots 0 0 0 1 2 2 2
  spline S229 degree 2 poles (-3.2103, -8.4531) (-3.1725, -8.4715) (-3.0793, -8.4987) (-3.0298, -8.4987) knots 0 0 0 1 2 2 2
  spline S230 degree 2 poles (-3.0298, -8.4987) (-2.9939, -8.4987) (-2.9114, -8.4822) (-2.8919, -8.4686) knots 0 0 0 1 2 2 2
  spline S231 degree 2 poles (-2.8919, -8.4686) (-2.8638, -8.4502) (-2.8386, -8.4084) (-2.8386, -8.3657) knots 0 0 0 1 2 2 2
  spline S232 degree 2 poles (-2.8386, -8.3657) (-2.8386, -8.3123) (-2.8968, -8.257) (-2.9715, -8.2385) knots 0 0 0 1 2 2 2
  spline S233 degree 2 poles (-2.9715, -8.2385) (-3.0007, -8.2317) (-3.0938, -8.2123) (-3.1336, -8.2017) knots 0 0 0 1 2 2 2
  spline S234 degree 2 poles (-3.1336, -8.2017) (-3.2365, -8.1716) (-3.3297, -8.0473) (-3.3297, -7.959) knots 0 0 0 1 2 2 2
  spline S235 degree 2 poles (-3.3297, -7.959) (-3.3297, -7.8367) (-3.1463, -7.6843) (-2.9948, -7.6843) knots 0 0 0 1 2 2 2
  spline S236 degree 2 poles (-2.9948, -7.6843) (-2.9201, -7.6843) (-2.7687, -7.7211) (-2.7172, -7.7493) knots 0 0 0 1 2 2 2
  line L171 (-2.7172, -7.7493) -> (-2.7172, -7.9114)
  line L172 (-2.7172, -7.9114) -> (-2.725, -7.9114)
  spline S237 degree 2 poles (-2.725, -7.9114) (-2.7832, -7.8648) (-2.9249, -7.8114) (-2.9977, -7.8114) knots 0 0 0 1 2 2 2
  spline S238 degree 2 poles (-2.9977, -7.8114) (-3.0725, -7.8114) (-3.1754, -7.8745) (-3.1754, -7.9376) knots 0 0 0 1 2 2 2
  spline S239 degree 2 poles (-3.1754, -7.9376) (-3.1754, -7.9949) (-3.1142, -8.0502) (-3.0463, -8.0677) knots 0 0 0 1 2 2 2
  spline S240 degree 2 poles (-3.0463, -8.0677) (-3.0133, -8.0764) (-2.9298, -8.0939) (-2.8842, -8.1046) knots 0 0 0 1 2 2 2
  spline S241 degree 2 poles (-2.8842, -8.1046) (-2.7852, -8.1298) (-2.6842, -8.2453) (-2.6842, -8.3453) knots 0 0 0 1 2 2 2
  spline S242 degree 2 poles (-2.6842, -8.3453) (-2.6842, -8.4036) (-2.7298, -8.5065) (-2.7745, -8.5443) knots 0 0 0 1 2 2 2
  spline S243 degree 2 poles (-2.7745, -8.5443) (-2.822, -8.5841) (-2.9434, -8.6259) (-3.0356, -8.6259) knots 0 0 0 1 2 2 2
  line L173 (-2.2513, -8.3754) -> (-2.4765, -8.9025)
  line L174 (-2.4765, -8.9025) -> (-2.5939, -8.9025)
  line L175 (-2.5939, -8.9025) -> (-2.4522, -8.3754)
  line L176 (-2.4522, -8.3754) -> (-2.2513, -8.3754)
  spline S244 degree 2 poles (-1.0505, -8.6259) (-1.167, -8.6259) (-1.364, -8.5472) (-1.4359, -8.4686) knots 0 0 0 1 2 2 2
  spline S245 degree 2 poles (-1.4359, -8.4686) (-1.5077, -8.3909) (-1.5863, -8.158) (-1.5863, -8.0065) knots 0 0 0 1 2 2 2
  spline S246 degree 2 poles (-1.5863, -8.0065) (-1.5863, -7.8561) (-1.5096, -7.6328) (-1.4368, -7.5503) knots 0 0 0 1 2 2 2
  spline S247 degree 2 poles (-1.4368, -7.5503) (-1.365, -7.4697) (-1.1689, -7.3853) (-1.0476, -7.3853) knots 0 0 0 1 2 2 2
  spline S248 degree 2 poles (-1.0476, -7.3853) (-0.9874, -7.3853) (-0.8816, -7.4028) (-0.8369, -7.4163) knots 0 0 0 1 2 2 2
  spline S249 degree 2 poles (-0.8369, -7.4163) (-0.7981, -7.429) (-0.7175, -7.4649) (-0.6777, -7.4862) knots 0 0 0 1 2 2 2
  line L177 (-0.6777, -7.4862) -> (-0.6777, -7.6784)
  line L178 (-0.6777, -7.6784) -> (-0.6904, -7.6784)
  spline S250 degree 2 poles (-0.6904, -7.6784) (-0.7117, -7.659) (-0.7777, -7.6047) (-0.8253, -7.5785) knots 0 0 0 1 2 2 2
  spline S251 degree 2 poles (-0.8253, -7.5785) (-0.8709, -7.5532) (-0.9787, -7.5212) (-1.0485, -7.5212) knots 0 0 0 1 2 2 2
  spline S252 degree 2 poles (-1.0485, -7.5212) (-1.1252, -7.5212) (-1.2621, -7.5843) (-1.3136, -7.6445) knots 0 0 0 1 2 2 2
  spline S253 degree 2 poles (-1.3136, -7.6445) (-1.364, -7.7056) (-1.4203, -7.891) (-1.4203, -8.0065) knots 0 0 0 1 2 2 2
  spline S254 degree 2 poles (-1.4203, -8.0065) (-1.4203, -8.1298) (-1.3611, -8.3075) (-1.3097, -8.3686) knots 0 0 0 1 2 2 2
  spline S255 degree 2 poles (-1.3097, -8.3686) (-1.2592, -8.4278) (-1.1243, -8.488) (-1.0485, -8.488) knots 0 0 0 1 2 2 2
  spline S256 degree 2 poles (-1.0485, -8.488) (-0.9796, -8.488) (-0.8622, -8.454) (-0.8165, -8.4288) knots 0 0 0 1 2 2 2
  spline S257 degree 2 poles (-0.8165, -8.4288) (-0.7729, -8.4036) (-0.7078, -8.3511) (-0.6894, -8.3327) knots 0 0 0 1 2 2 2
  line L179 (-0.6894, -8.3327) -> (-0.6777, -8.3327)
  line L180 (-0.6777, -8.3327) -> (-0.6777, -8.523)
  spline S258 degree 2 poles (-0.6777, -8.523) (-0.7175, -8.5414) (-0.7874, -8.5754) (-0.8369, -8.5909) knots 0 0 0 1 2 2 2
  spline S259 degree 2 poles (-0.8369, -8.5909) (-0.8894, -8.6084) (-0.9787, -8.6259) (-1.0505, -8.6259) knots 0 0 0 1 2 2 2
  spline S260 degree 2 poles (0.1979, -8.1551) (0.1979, -8.3822) (-0.0206, -8.6297) (-0.2031, -8.6297) knots 0 0 0 1 2 2 2
  spline S261 degree 2 poles (-0.2031, -8.6297) (-0.3904, -8.6297) (-0.6049, -8.3744) (-0.6049, -8.1551) knots 0 0 0 1 2 2 2
  spline S262 degree 2 poles (-0.6049, -8.1551) (-0.6049, -7.9299) (-0.3836, -7.6804) (-0.2031, -7.6804) knots 0 0 0 1 2 2 2
  spline S263 degree 2 poles (-0.2031, -7.6804) (-0.0206, -7.6804) (0.1979, -7.9289) (0.1979, -8.1551) knots 0 0 0 1 2 2 2
  spline S264 degree 2 poles (0.0416, -8.1551) (0.0416, -7.9803) (-0.0856, -7.8105) (-0.2031, -7.8105) knots 0 0 0 1 2 2 2
  spline S265 degree 2 poles (-0.2031, -7.8105) (-0.3205, -7.8105) (-0.4486, -7.9803) (-0.4486, -8.1551) knots 0 0 0 1 2 2 2
  spline S266 degree 2 poles (-0.4486, -8.1551) (-0.4486, -8.3249) (-0.3205, -8.4997) (-0.2031, -8.4997) knots 0 0 0 1 2 2 2
  spline S267 degree 2 poles (-0.2031, -8.4997) (-0.0866, -8.4997) (0.0416, -8.3278) (0.0416, -8.1551) knots 0 0 0 1 2 2 2
  line L181 (0.5881, -8.6045) -> (0.3959, -8.6045)
  line L182 (0.3959, -8.6045) -> (0.3959, -8.3754)
  line L183 (0.3959, -8.3754) -> (0.5881, -8.3754)
  line L184 (0.5881, -8.3754) -> (0.5881, -8.6045)
  line L185 (2.0723, -8.6045) -> (1.3782, -8.6045)
  line L186 (1.3782, -8.6045) -> (1.3782, -7.4066)
  line L187 (1.3782, -7.4066) -> (1.5374, -7.4066)
  line L188 (1.5374, -7.4066) -> (1.5374, -8.4628)
  line L189 (1.5374, -8.4628) -> (2.0723, -8.4628)
  line L190 (2.0723, -8.4628) -> (2.0723, -8.6045)
  spline S268 degree 2 poles (2.4577, -8.622) (2.3344, -8.622) (2.1956, -8.4812) (2.1956, -8.3288) knots 0 0 0 1 2 2 2
  line L191 (2.1956, -8.3288) -> (2.1956, -7.8308)
  line L192 (2.1956, -7.8308) -> (2.0937, -7.8308)
  line L193 (2.0937, -7.8308) -> (2.0937, -7.7056)
  line L194 (2.0937, -7.7056) -> (2.1956, -7.7056)
  line L195 (2.1956, -7.7056) -> (2.1956, -7.4474)
  line L196 (2.1956, -7.4474) -> (2.347, -7.4474)
  line L197 (2.347, -7.4474) -> (2.347, -7.7056)
  line L198 (2.347, -7.7056) -> (2.6256, -7.7056)
  line L199 (2.6256, -7.7056) -> (2.6256, -7.8308)
  line L200 (2.6256, -7.8308) -> (2.347, -7.8308)
  line L201 (2.347, -7.8308) -> (2.347, -8.2589)
  spline S269 degree 2 poles (2.347, -8.2589) (2.347, -8.3269) (2.3519, -8.4016) (2.3684, -8.4337) knots 0 0 0 1 2 2 2
  spline S270 degree 2 poles (2.3684, -8.4337) (2.382, -8.4618) (2.4431, -8.49) (2.4955, -8.49) knots 0 0 0 1 2 2 2
  spline S271 degree 2 poles (2.4955, -8.49) (2.5324, -8.49) (2.6013, -8.4676) (2.6169, -8.4608) knots 0 0 0 1 2 2 2
  line L202 (2.6169, -8.4608) -> (2.6256, -8.4608)
  line L203 (2.6256, -8.4608) -> (2.6256, -8.5967)
  spline S272 degree 2 poles (2.6256, -8.5967) (2.5829, -8.6084) (2.4955, -8.622) (2.4577, -8.622) knots 0 0 0 1 2 2 2
  line L204 (3.4284, -8.6045) -> (3.277, -8.6045)
  line L205 (3.277, -8.6045) -> (3.277, -8.5133)
  spline S273 degree 2 poles (3.277, -8.5133) (3.242, -8.5424) (3.1906, -8.5812) (3.1556, -8.5977) knots 0 0 0 1 2 2 2
  spline S274 degree 2 poles (3.1556, -8.5977) (3.1236, -8.6132) (3.0547, -8.6297) (3.009, -8.6297) knots 0 0 0 1 2 2 2
  spline S275 degree 2 poles (3.009, -8.6297) (2.9353, -8.6297) (2.811, -8.5686) (2.7673, -8.5094) knots 0 0 0 1 2 2 2
  spline S276 degree 2 poles (2.7673, -8.5094) (2.7237, -8.4502) (2.6751, -8.2754) (2.6751, -8.1619) knots 0 0 0 1 2 2 2
  spline S277 degree 2 poles (2.6751, -8.1619) (2.6751, -8.0434) (2.7363, -7.8706) (2.7897, -7.8056) knots 0 0 0 1 2 2 2
  spline S278 degree 2 poles (2.7897, -7.8056) (2.8392, -7.7474) (2.978, -7.6804) (3.0547, -7.6804) knots 0 0 0 1 2 2 2
  spline S279 degree 2 poles (3.0547, -7.6804) (3.1216, -7.6804) (3.2216, -7.7105) (3.277, -7.7415) knots 0 0 0 1 2 2 2
  line L206 (3.277, -7.7415) -> (3.277, -7.3532)
  line L207 (3.277, -7.3532) -> (3.4284, -7.3532)
  line L208 (3.4284, -7.3532) -> (3.4284, -8.6045)
  line L209 (3.277, -8.3861) -> (3.277, -7.8668)
  spline S280 degree 2 poles (3.277, -7.8668) (3.2207, -7.8396) (3.1314, -7.8192) (3.0799, -7.8192) knots 0 0 0 1 2 2 2
  spline S281 degree 2 poles (3.0799, -7.8192) (2.9634, -7.8192) (2.8314, -7.9939) (2.8314, -8.1589) knots 0 0 0 1 2 2 2
  spline S282 degree 2 poles (2.8314, -8.1589) (2.8314, -8.3181) (2.9324, -8.4861) (3.044, -8.4861) knots 0 0 0 1 2 2 2
  spline S283 degree 2 poles (3.044, -8.4861) (3.1032, -8.4861) (3.2236, -8.4317) (3.277, -8.3861) knots 0 0 0 1 2 2 2
  line L210 (3.8827, -8.6045) -> (3.6905, -8.6045)
  line L211 (3.6905, -8.6045) -> (3.6905, -8.3754)
  line L212 (3.6905, -8.3754) -> (3.8827, -8.3754)
  line L213 (3.8827, -8.3754) -> (3.8827, -8.6045)
  point P0 (0, 0)
  constraints: 2 other
emboss "Emboss1" sketch "Sketch2" operation add depth 0.5 direction (0, 0, -1)
fillet "Fillet1" radius 1 4 edges at (0, -10.16, 2) (-25.4, 0, 2) (0, 10.16, 2) (25.4, 0, 2)
body "Solid1"
